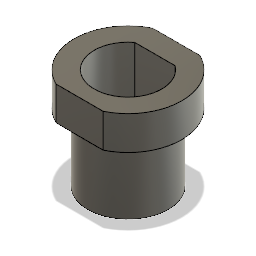
Anel_Helice (Autodesk Fusion 360 design; units mm, degrees)
Autodesk Fusion 360 part; units mm, degrees
sketch "Sketch1" plane through (0, 0, 0) normal (0, 1, 0) x (1, 0, 0)
  arc A0 (-1.5, 2) -> (1.5, 2) centre (0, 0) ccw
  line L0 (1.5, 2) -> (-1.5, 2)
  circle A1 centre (0, 0) radius 3
  dimension "d2" = 3
  dimension "d3" = 2.5
  dimension "d4" = 6
  constraint coincident A0.centre A1.centre
  constraint horizontal A0.start A0.end
  constraint concentric A0 A1
  measures "d2" distance of A0.start A0.end
  measures "d3" radius of A0
  measures "d4" diameter of A1
extrude "Extrude1" add sketch "Sketch1" along normal blind 5
sketch "Sketch2" plane through (0, 5, 0) normal (0, 1, 0) x (-1, 0, 0)
  arc A0 (1.5, -2) -> (-1.5, -2) centre (0, 0) ccw
  line L0 (-1.5, -2) -> (1.5, -2)
  arc A1 (1.75, -3.5969) -> (1.75, 3.5969) centre (0, 0) ccw
  arc A2 (-1.75, 3.5969) -> (-1.75, -3.5969) centre (0, 0) ccw
  line L1 (-1.75, -3.5969) -> (1.75, -3.5969)
  line L2 (1.75, 3.5969) -> (-1.75, 3.5969)
  dimension "d7" = 3
  dimension "d8" = 2.5
  dimension "d9" = 4
  dimension "d10" = 4
  dimension "d11" = 3.5
  dimension "d12" = 3.5
  constraint coincident A0.centre A1.centre
  constraint horizontal L0
  constraint horizontal A1.start A2.end
  constraint horizontal A1.end A2.start
  measures "d7" distance of A0.start A0.end
  measures "d8" radius of A0
  measures "d9" radius of A2
  measures "d10" radius of A1
  measures "d11" distance of A1.end A2.start
  measures "d12" distance of A1.start A2.end
extrude "Extrude2" add sketch "Sketch2" along normal blind 2.5
